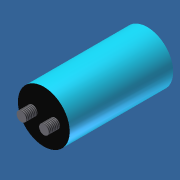
# Autodesk Inventor part: Cap
Saved by Autodesk Inventor 2012 (Build 160160000, 160)
## iProperties
Created: 2012-03-25
Part Number: Cap
Material: Default
Document SubType Name: Modeling
Designer: Edward
Density: 1 g/cm^3
Author: Edward
Autodesk Inventor part; units mm, degrees
ref_plane "YZ Plane" through (0, 0, 0) normal (1, 0, 0) x (0, 1, 0)
ref_plane "XZ Plane" through (0, 0, 0) normal (0, 1, 0) x (-1, 0, 0)
ref_plane "XY Plane" through (0, 0, 0) normal (0, 0, 1) x (1, 0, 0)
sketch "Sketch1" plane through (0, 0, 0) normal (0, 0, 1) x (1, 0, 0)
  circle A0 centre (0, 0) radius 25.4
  dimension "d0" = 50.8
  constraints: 1 centre point, 1 coincident
  measures "d0" diameter of A0
extrude "Can" add sketch "Sketch1" along normal blind 101.6
sketch "Sketch2" plane through (0, 0, 101.6) normal (0, 0, 1) x (1, 0, 0)
  circle A0 centre (0, 0) radius 25.4 projected
  circle A1 centre (-11.049, 0) radius 4.7625
  circle A2 centre (11.049, 0) radius 4.7625
  dimension "d3" = 9.525
  dimension "d4" = 22.098
  dimension "d5" = 11.049
  constraints: 2 centre point, 2 horizontal alignment, 1 equal radius
  measures "d3" diameter of A2
  measures "d4" distance of A1.centre A2.centre
  measures "d5" distance of A0.centre A2.centre
extrude "Studs" add sketch "Sketch2" along normal blind 10.922 contours A1 | A2
thread "Stud 1" size "3/8-16 UNC" class "2A" standard "ANSI Unified Screw Threads" full length
thread "Stud 2" size "3/8-16 UNC" class "2A" standard "ANSI Unified Screw Threads" full length
equation "\"d5\" = 0.5 * d4"
body "Solid1"
